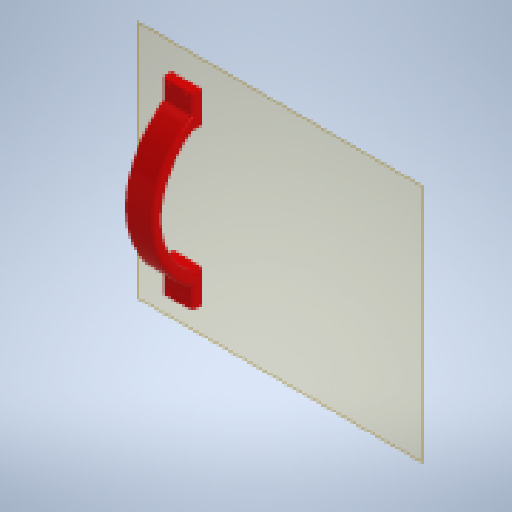
# Autodesk Inventor part: ручка
Saved by Autodesk Inventor 2024.2 (Build 282272000, 272)
## iProperties
Created: 2026-01-10
Part Number: ручка
Material: Типовые
Document SubType Name: Modeling
Designer: katya_notebook
Density: 1 g/cm^3
Appearance: Красный
Author: katya_notebook
Autodesk Inventor part; units mm, degrees
ref_plane "YZ Plane" through (0, 0, 0) normal (1, 0, 0) x (0, 1, 0)
ref_plane "XZ Plane" through (0, 0, 0) normal (0, 1, 0) x (-1, 0, 0)
ref_plane "XY Plane" through (0, 0, 0) normal (0, 0, 1) x (1, 0, 0)
ref_plane "РабПлоскость1" through (0, 0, 0) normal (0, 0, 1) x (1, 0, 0)
sketch "Эскиз1" plane through (0, 0, 0) normal (0, 0, 1) x (1, 0, 0)
  circle A0 centre (-106.5237, 94.25) radius 1.75 projected
  circle A1 centre (-88.5237, 94.25) radius 1.75 projected
  circle A2 centre (-106.5237, -94.25) radius 1.75 projected
  circle A3 centre (-88.5237, -94.25) radius 1.75 projected
  line L0 (-127, -97.5) -> (-62.5237, -97.5) projected
  line L1 (-62.5237, 97.5) -> (-127, 97.5) projected
  line L2 (-127, 97.5) -> (-69.1452, 97.5)
  line L3 (-69.1452, 97.5) -> (-69.1452, 77.5)
  line L4 (-69.1452, 77.5) -> (-127, 77.5)
  line L5 (-127, 77.5) -> (-127, 97.5)
  line L6 (0, 0) -> (-182.8983, 0)
  circle A4 centre (-106.5237, -94.25) radius 1.75
  circle A5 centre (-88.5237, -94.25) radius 1.75
  line L7 (-62.5237, -97.5) -> (-127, -97.5)
  line L8 (-127, -97.5) -> (-69.1452, -97.5)
  line L9 (-69.1452, -97.5) -> (-69.1452, -77.5)
  line L10 (-69.1452, -77.5) -> (-127, -77.5)
  line L11 (-127, -77.5) -> (-127, -97.5)
  line L12 (-81.0199, 97.5) -> (-81.0199, -97.5)
  line L13 (-113.2834, -97.5) -> (-113.2834, 97.5)
  point P0 (-113.2834, -77.5)
  point P1 (-81.0199, -77.5)
  point P2 (-113.2834, 77.5)
  point P3 (-81.0199, 77.5)
  dimension "d0" = 20
  constraints: 24 end point, 5 symmetric about line, 4 point on line, 3 perpendicular, 2 centre point, 2 horizontal, 2 parallel, 2 other
  measures "d0" distance of L4.end L1.end
extrude "Выдавливание1" add sketch "Эскиз1" along normal blind 10 contours L13 L10 L12 L0 | L13 L1 L12 L4
sketch "Эскиз3" plane through (-113.2834, -97.5, 0) normal (-1, 0, 0) x (0, 0, 1)
  line L0 (0, 175) -> (0, 160)
  line L1 (0, 160) -> (10, 160)
  line L2 (10, 160) -> (10, 175)
  line L3 (10, 175) -> (0, 175)
  line L4 (0, 20) -> (10, 20) projected
  line L5 (10, 20) -> (0, 20)
  line L6 (0, 20) -> (0, 35)
  line L7 (0, 35) -> (10, 35)
  line L8 (10, 35) -> (10, 20)
  arc A0 (10, 20) -> (10, 175) centre (-44.9432, 97.5) ccw
  arc A1 (10, 35) -> (10, 160) centre (-39.9375, 97.5) ccw
  point P0 (0, 97.5)
  dimension "d10" = 15
  dimension "d11" = 15
  dimension "d12" = 95
  dimension "d13" = 80
  dimension "d16" = 10
  constraints: 16 end point, 4 point on circle, 3 perpendicular, 2 centre point, 2 parallel, 1 horizontal, 1 vertical
  measures "d10" distance of L0.start L0.end
  measures "d11" distance of L5.end L6.end
  measures "d12" radius of A0
  measures "d13" radius of A1
  measures "d16" distance of L6.end L7.end
extrude "Выдавливание3" add sketch "Эскиз3" against normal up to surface (32.2635 mm away)
fillet "Сопряжение1" radius 4 8 edges at (-113.2834, 0, 50.0568) (-113.2834, 0, 40.0625) (-81.0199, 0, 50.0568) (-81.0199, 0, 40.0625) (-113.2834, 62.5, 5) (-113.2834, -62.5, 5) (-81.0199, -62.5, 5) (-81.0199, 62.5, 5)
fillet "Сопряжение2" radius 4 8 edges at (-113.2834, -75.0207, 10) (-113.2834, -87.5, 10) (-81.0199, -75.0207, 10) (-81.0199, -87.5, 10) (-81.0199, 75.0207, 10) (-81.0199, 87.5, 10) (-113.2834, 75.0207, 10) (-113.2834, 87.5, 10)
